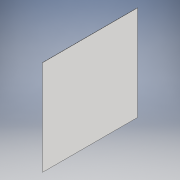
# Autodesk Inventor part: White Board
Saved by Autodesk Inventor 2019 (Build 230136000, 136)
## iProperties
Created: 2019-01-19
Part Number: White Board
Material: Generic
Document SubType Name: Modeling
Designer: nxgam
Density: 1 g/cm^3
Appearance: Default(1)
Author: nxgam
Autodesk Inventor part; units mm, degrees
ref_plane "YZ Plane" through (0, 0, 0) normal (1, 0, 0) x (0, 1, 0)
ref_plane "XZ Plane" through (0, 0, 0) normal (0, 1, 0) x (-1, 0, 0)
ref_plane "XY Plane" through (0, 0, 0) normal (0, 0, 1) x (1, 0, 0)
sketch "Sketch1" plane through (0, 0, 0) normal (1, 0, 0) x (0, 1, 0)
  line L0 (-609.6, 609.6) -> (609.6, 609.6)
  line L1 (609.6, 609.6) -> (609.6, -609.6)
  line L2 (609.6, -609.6) -> (-609.6, -609.6)
  line L3 (-609.6, -609.6) -> (-609.6, 609.6)
  line L4 (-609.6, 609.6) -> (609.6, -609.6) construction
  line L5 (609.6, 609.6) -> (-609.6, -609.6) construction
  point P0 (0, 0)
  dimension "d0" = 1219.2
  dimension "d1" = 1219.2
  constraints: 12 end point, 2 midpoint, 2 parallel, 1 horizontal, 1 perpendicular
  measures "d0" distance of L1.end L2.end
  measures "d1" distance of L0.end L1.end
extrude "Extrusion1" add sketch "Sketch1" along normal blind 2.54
body "Solid1"
